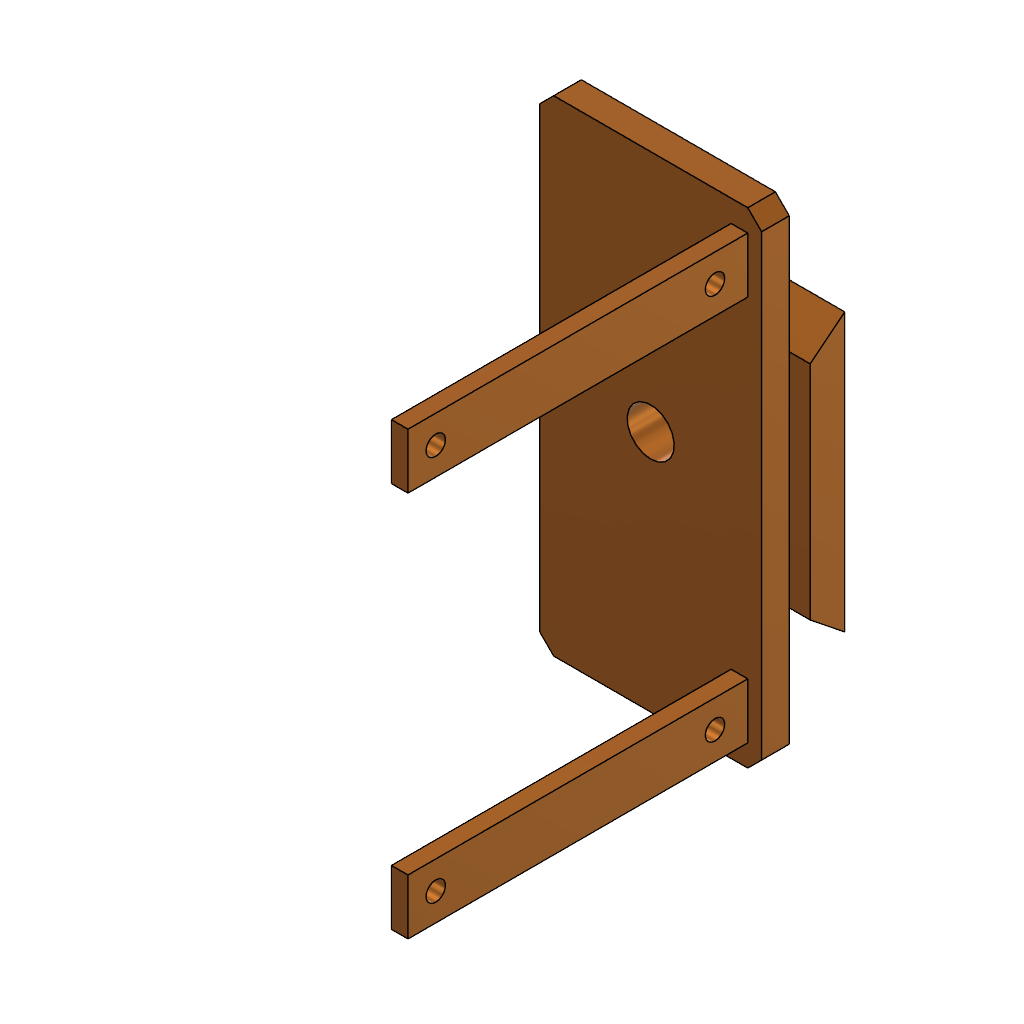
camera_plate_four_screw (Autodesk Fusion 360 design; units mm, degrees)
part number: 2026-10-03-13-24-09-908
Autodesk Fusion 360 part; units mm, degrees
ref_plane "工作平面1" through (0, 0, 12.3) normal (0, 0, 1) x (1, 0, 0)
sketch "草图1" plane through (0, 0, 12.3) normal (0, 0, 1) x (1, 0, 0)
  line L0 (-33, -16) -> (33, -16)
  line L1 (33, -16) -> (35, -14)
  line L2 (35, -14) -> (35, 14)
  line L3 (35, 14) -> (33, 16)
  line L4 (33, 16) -> (-33, 16)
  line L5 (-33, 16) -> (-35, 14)
  line L6 (-35, 14) -> (-35, -14)
  line L7 (-35, -14) -> (-33, -16)
extrude "70 x 32 camera support plate" add sketch "草图1" along normal blind 4
ref_plane "工作平面2" through (0, 0, 7.3) normal (0, 0, 1) x (1, 0, 0)
sketch "草图2" plane through (0, 0, 7.3) normal (0, 0, 1) x (1, 0, 0)
  line L0 (-20, -19) -> (20, -19)
  line L1 (20, -19) -> (20, 19)
  line L2 (20, 19) -> (-20, 19)
  line L3 (-20, 19) -> (-20, -19)
ref_plane "工作平面3" through (0, 0, 12.3) normal (0, 0, 1) x (1, 0, 0)
sketch "草图3" plane through (0, 0, 12.3) normal (0, 0, 1) x (1, 0, 0)
  line L0 (-16, -19) -> (16, -19)
  line L1 (16, -19) -> (16, 19)
  line L2 (16, 19) -> (-16, 19)
  line L3 (-16, 19) -> (-16, -19)
loft "40 to 32 mm male dovetail" add profiles "草图2", "草图3" section 1 section 2
ref_plane "工作平面4" through (0, 0, 7.3) normal (0, 0, 1) x (1, 0, 0)
sketch "草图4" plane through (0, 0, 7.3) normal (0, 0, 1) x (1, 0, 0)
  circle A0 centre (0, 0) radius 3.4
extrude "1/4 inch metal screw clearance 6.8 mm" cut sketch "草图4" along normal blind 9
ref_plane "工作平面5" through (0, 0, 7.3) normal (0, 0, 1) x (1, 0, 0)
sketch "草图5" plane through (0, 0, 7.3) normal (0, 0, 1) x (1, 0, 0)
  circle A0 centre (0, 0) radius 7
extrude "14 x 3.5 mm screw head recess" cut sketch "草图5" along normal blind 3.5
ref_plane "工作平面6" through (0, 0, 16.3) normal (0, 0, 1) x (1, 0, 0)
sketch "草图6" plane through (0, 0, 16.3) normal (0, 0, 1) x (1, 0, 0)
  line L0 (-31.8391, -14.0004) -> (-23.8391, -14.0004)
  line L1 (-23.8391, -14.0004) -> (-23.8391, -11.6004)
  line L2 (-23.8391, -11.6004) -> (-31.8391, -11.6004)
  line L3 (-31.8391, -11.6004) -> (-31.8391, -14.0004)
extrude "Front four screw support column" add sketch "草图6" along normal blind 49
ref_plane "工作平面7" through (0, 0, 16.3) normal (0, 0, 1) x (1, 0, 0)
sketch "草图7" plane through (0, 0, 16.3) normal (0, 0, 1) x (1, 0, 0)
  line L0 (23.8391, -14.0004) -> (31.8391, -14.0004)
  line L1 (31.8391, -14.0004) -> (31.8391, -11.6004)
  line L2 (31.8391, -11.6004) -> (23.839, -11.6004)
  line L3 (23.8391, -11.6004) -> (23.8391, -14.0004)
extrude "Front four screw support column (1)" add sketch "草图7" along normal blind 49
ref_plane "工作平面8" through (0, 14.0004, 0) normal (0, 1, 0) x (0, 0, 1)
sketch "草图8" plane through (0, 14.0004, 0) normal (0, 1, 0) x (1, 0, 0)
  circle A0 through (-26.4391, -21.023, -28.0009) (-28.5391, -19.8105, -28.0009) (-28.5391, -22.2354, -28.0009)
  circle A1 through (-26.4391, -61.297, -28.0009) (-28.5391, -60.0846, -28.0009) (-28.5391, -62.5095, -28.0009)
  circle A2 through (29.2391, -21.023, -28.0009) (27.1391, -19.8105, -28.0009) (27.139, -22.2354, -28.0009)
  circle A3 through (29.2391, -61.297, -28.0009) (27.1391, -60.0846, -28.0009) (27.139, -62.5095, -28.0009)
extrude "Four 2.8 mm auxiliary screw clearances" cut sketch "草图8" along normal blind 2.4 contours A0 | A1 | A2 | A3 in plane through (0, -14.0005, 0) normal (0, 1, 0)
move_body "Align camera long edge with gimbal arm - 90 degrees" bodies 1 to x (0, 1, 0) y (-1, 0, 0) z (0, 0, 1) at (0, 0, 0)
named bodies: "Camera_plate_1_4_four_screw_v2"
